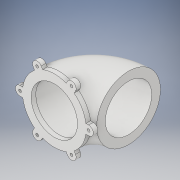
# Autodesk Inventor part: TARM01
Saved by Autodesk Inventor 2017 (Build 210142000, 142)
## iProperties
Created: 2018-10-11
Part Number: TARM01
Material: ABS Plastic
Document SubType Name: Modeling
Designer: Zach
Density: 1.06 g/cm^3
Appearance: Smooth - White
Author: Zach
Autodesk Inventor part; units mm, degrees
ref_plane "YZ Plane" through (0, 0, 0) normal (1, 0, 0) x (0, 1, 0)
ref_plane "XZ Plane" through (0, 0, 0) normal (0, 1, 0) x (-1, 0, 0)
ref_plane "XY Plane" through (0, 0, 0) normal (0, 0, 1) x (1, 0, 0)
sketch "Sketch1" plane through (0, 0, 0) normal (0, 0, 1) x (1, 0, 0)
  circle A0 centre (0, 0) radius 68.75
  circle A1 centre (74, 0) radius 3
  circle A2 centre (37, 64.0859) radius 3
  circle A3 centre (-37, 64.0859) radius 3
  circle A4 centre (-74, 0) radius 3
  circle A5 centre (-37, -64.0859) radius 3
  circle A6 centre (37, -64.0859) radius 3
  circle A7 centre (74, 0) radius 10
  line L0 (74, 10) -> (68.0188, 10)
  line L1 (74, -10) -> (68.0188, -10)
  line L2 (68.0188, 10) -> (68.0188, -10)
  line L3 (28.3397, 69.0859) -> (25.3492, 63.906)
  line L4 (25.3492, 63.906) -> (42.6697, 53.906)
  line L5 (45.6603, 59.0859) -> (42.6697, 53.906)
  circle A8 centre (37, 64.0859) radius 10
  line L6 (-45.6603, 59.0859) -> (-42.6697, 53.906)
  line L7 (-42.6697, 53.906) -> (-25.3492, 63.906)
  line L8 (-28.3397, 69.0859) -> (-25.3492, 63.906)
  circle A9 centre (-37, 64.0859) radius 10
  line L9 (-74, -10) -> (-68.0188, -10)
  line L10 (-68.0188, -10) -> (-68.0188, 10)
  line L11 (-74, 10) -> (-68.0188, 10)
  circle A10 centre (-74, 0) radius 10
  line L12 (-28.3397, -69.0859) -> (-25.3492, -63.906)
  line L13 (-25.3492, -63.906) -> (-42.6697, -53.906)
  line L14 (-45.6603, -59.0859) -> (-42.6697, -53.906)
  circle A11 centre (-37, -64.0859) radius 10
  line L15 (45.6603, -59.0859) -> (42.6697, -53.906)
  line L16 (42.6697, -53.906) -> (25.3492, -63.906)
  line L17 (28.3397, -69.0859) -> (25.3492, -63.906)
  circle A12 centre (37, -64.0859) radius 10
  circle A13 centre (0, 0) radius 50
  dimension "d0" = 137.5
  dimension "d1" = 6
  dimension "d2" = 74
  dimension "d5" = 360
  dimension "d7" = 20
  dimension "d10" = 360
  dimension "d12" = 100
  constraints: 36 end point, 14 centre point, 14 point on circle, 5 coincident, 2 tangent, 1 horizontal, 1 horizontal alignment, 1 parallel, 1 vertical, 72 other
  measures "d0" diameter of A0
  measures "d1" diameter of A1
  measures "d2" distance of point (0, 0) A1.centre
  measures "d7" diameter of A7
  measures "d12" diameter of A13
extrude "Extrusion1" add sketch "Sketch1" along normal blind 10
sketch "Sketch2" plane through (0, 0, 0) normal (0, 0, -1) x (-1, 0, 0)
  line L0 (68.0188, 10) -> (74, 10) projected
  circle A0 centre (0, 0) radius 68.75
  circle A1 centre (0, 0) radius 50 projected
  constraints: 1 coincident, 3 other
sketch "Sketch3" plane through (0, 0, 0) normal (0, 1, 0) x (-1, 0, 0)
  arc A0 (-75, -75) -> (0, 0) centre (-75, 0) ccw
  line L0 (0, 0) -> (0, 44.6064) construction
  line L1 (-75, -75) -> (-105.1749, -75) construction
  dimension "d15" = 75
  constraints: 4 end point, 2 point on circle, 2 tangent, 1 centre point, 1 horizontal, 1 vertical
  measures "d15" radius of A0
sweep "Sweep1" add profiles "Sketch2" path "Sketch3"
body "Solid1"
